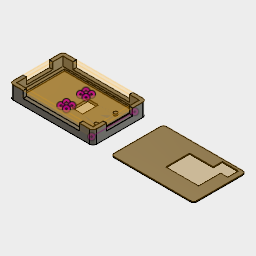
Tstat_case (Autodesk Fusion 360 design; units mm, degrees)
Autodesk Fusion 360 part; units mm, degrees
sketch "Sketch1" plane through (0, 0, 0) normal (0, 1, 0) x (1, 0, 0)
  line L0 (76, 53) -> (-76, 53)
  line L1 (-83, 46) -> (-83, -46)
  line L2 (-76, -53) -> (76, -53)
  line L3 (83, -46) -> (83, 46)
  line L4 (83, 53) -> (-83, -53) construction
  line L5 (-83, 53) -> (83, -53) construction
  line L6 (-76, 46) -> (76, 46)
  line L7 (76, 46) -> (76, -46)
  line L8 (76, -46) -> (-76, -46)
  line L9 (-76, -46) -> (-76, 46)
  line L10 (-76, 46) -> (76, -46) construction
  line L11 (76, 46) -> (-76, -46) construction
  arc A0 (-76, 53) -> (-83, 46) centre (-76, 46) ccw
  arc A1 (-83, -46) -> (-76, -53) centre (-76, -46) ccw
  arc A2 (83, 46) -> (76, 53) centre (76, 46) ccw
  arc A3 (76, -53) -> (83, -46) centre (76, -46) ccw
  dimension "d1" = 166
  dimension "d2" = 106
  dimension "d3" = 152
  dimension "d4" = 92
  dimension "d5" = 7
  dimension "d6" = 7
  dimension "d7" = 7
  dimension "d8" = 7
  constraint perpendicular L0 L1
  constraint parallel L0 L2
  constraint parallel L1 L3
  constraint horizontal L0
  constraint coincident L4
  constraint coincident L5
  constraint perpendicular L6 L7
  constraint parallel L6 L8
  constraint parallel L7 L9
  constraint horizontal L6
  constraint coincident L10
  constraint coincident L11
  constraint tangent L0 A0
  constraint tangent L1 A0
  constraint tangent L1 A1
  constraint tangent L2 A1
  constraint tangent L0 A2
  constraint tangent L3 A2
  constraint tangent L3 A3
  constraint tangent L2 A3
  measures "d5" radius of A0
  measures "d6" radius of A1
  measures "d7" radius of A2
  measures "d8" radius of A3
extrude "Extrude1" add sketch "Sketch1" along normal blind 5 contours L0 L1 L2 L3 A0 A1 A2 A3 | L6 L7 L8 L9 makes body 1
sketch "Sketch2" plane through (0, 5, 0) normal (0, 1, 0) x (-1, 0, 0)
  arc A0 (-76, 53) -> (-83, 46) centre (-76, 46) ccw
  line L0 (-83, 46) -> (-83, -46)
  arc A1 (-83, -46) -> (-76, -53) centre (-76, -46) ccw
  line L1 (-76, -53) -> (76, -53)
  arc A2 (76, -53) -> (83, -46) centre (76, -46) ccw
  line L2 (83, -46) -> (83, 46)
  arc A3 (83, 46) -> (76, 53) centre (76, 46) ccw
  line L3 (76, 53) -> (-76, 53)
  line L4 (-76, 46) -> (76, 46)
  line L5 (76, 46) -> (76, -46)
  line L6 (76, -46) -> (-76, -46)
  line L7 (-76, -46) -> (-76, 46)
  line L8 (-76, 46) -> (76, -46) construction
  line L9 (76, 46) -> (-76, -46) construction
  dimension "d11" = 152
  dimension "d12" = 92
  constraint perpendicular L4 L5
  constraint parallel L4 L6
  constraint parallel L5 L7
  constraint horizontal L4
  constraint coincident L8
  constraint coincident L9
extrude "Extrude2" add sketch "Sketch2" along normal blind 21.5 bodies 1
sketch "Sketch3" plane through (0, 5, 0) normal (0, 1, 0) x (-1, 0, 0)
  line L0 (76, -46) -> (76, 46)
  line L1 (76, 46) -> (-76, 46)
  line L2 (-76, 46) -> (-76, -46)
  line L3 (-76, -46) -> (76, -46)
  line L4 (70, -43) -> (-70, -43)
  line L5 (-70, -43) -> (-70, 43)
  line L6 (-70, 43) -> (70, 43)
  line L7 (70, 43) -> (70, -43)
  line L8 (70, -43) -> (-70, 43) construction
  line L9 (-70, -43) -> (70, 43) construction
  dimension "d15" = 140
  dimension "d16" = 86
  constraint perpendicular L4 L5
  constraint parallel L4 L6
  constraint parallel L5 L7
  constraint horizontal L4
  constraint coincident L8
  constraint coincident L9
extrude "Extrude3" add sketch "Sketch3" along normal blind 3.5 bodies 1
sketch "Sketch4" plane through (0, 5, 0) normal (0, 1, 0) x (-1, 0, 0)
  line L0 (-70, 43) -> (-70, -43)
  line L1 (-70, -43) -> (70, -43)
  line L2 (70, -43) -> (70, 43)
  line L3 (70, 43) -> (-70, 43)
  circle A0 centre (-55.85, -18.95) radius 3.45
  dimension "d19" = 6.9
  dimension "d20" = 14.15
  dimension "d21" = 24.05
  measures "d19" diameter of A0
  measures "d20" distance of L0
  measures "d21" distance of L1
extrude "Extrude4" add sketch "Sketch4" along normal blind 3.5 contours A0 bodies 1
sketch "Sketch5" plane through (0, 5, 0) normal (0, 1, 0) x (-1, 0, 0)
  circle A0 centre (-55.85, -18.95) radius 3.45
  line L0 (-70, 43) -> (-70, -43)
  line L1 (-70, -43) -> (70, -43)
  line L2 (70, -43) -> (70, 43)
  line L3 (70, 43) -> (-70, 43)
  line L4 (-1, -18.5) -> (-22, -18.5)
  line L5 (-22, -18.5) -> (-22, 12.5)
  line L6 (-22, 12.5) -> (-1, 12.5)
  line L7 (-1, 12.5) -> (-1, -18.5)
  line L8 (14, -30) -> (3, -30)
  line L9 (3, -30) -> (3, -19)
  line L10 (3, -19) -> (14, -19)
  line L11 (14, -19) -> (14, -30)
  line L12 (14, 9) -> (3, 9)
  line L13 (3, 9) -> (3, 20)
  line L14 (3, 20) -> (14, 20)
  line L15 (14, 20) -> (14, 9)
  dimension "d24" = 21
  dimension "d28" = 11
  dimension "d29" = 11
  dimension "d32" = 11
  dimension "d33" = 11
  dimension "d84" = 56
  dimension "d85" = 56
  dimension "d86" = 48
  dimension "d87" = 31
  dimension "d88" = 30.5
  dimension "d89" = 13
  dimension "d90" = 23
  constraint horizontal L4
  constraint vertical L5
  constraint horizontal L6
  constraint vertical L7
  constraint horizontal L8
  constraint vertical L9
  constraint horizontal L10
  constraint vertical L11
  constraint horizontal L12
  constraint vertical L13
  constraint horizontal L14
  constraint vertical L15
  measures "d84" distance of L2 L11
  measures "d85" distance of L2
  measures "d86" distance of L0 L5
  measures "d88" distance of L3 L6
  measures "d89" distance of L1
  measures "d90" distance of L3
extrude "Extrude5" cut sketch "Sketch5" against normal blind 5 contours L4 L5 L6 L7 bodies 1
extrude "Extrude11" add sketch "Sketch5" along normal blind 1 contours L8 L9 L10 L11 | L12 L13 L14 L15 bodies 1
sketch "Sketch6" plane through (0, 5, 0) normal (0, 1, 0) x (-1, 0, 0)
  line L0 (-22, -18.5) -> (-22, 12.5)
  line L1 (-22, 12.5) -> (-1, 12.5)
  line L2 (-1, 12.5) -> (-1, -18.5)
  line L3 (-1, -18.5) -> (-22, -18.5)
  circle A0 centre (-55.85, -18.95) radius 3.45
  line L4 (-70, 43) -> (-70, -43)
  line L5 (-70, -43) -> (70, -43)
  line L6 (70, -43) -> (70, 43)
  line L7 (70, 43) -> (-70, 43)
sketch "Sketch7" plane through (0, 5, 0) normal (0, 1, 0) x (-1, 0, 0)
  line L0 (-22, -18.5) -> (-22, 12.5)
  line L1 (-22, 12.5) -> (-1, 12.5)
  line L2 (-1, 12.5) -> (-1, -18.5)
  line L3 (-1, -18.5) -> (-22, -18.5)
  circle A0 centre (-55.85, -18.95) radius 3.45
  line L4 (-70, 43) -> (-70, -43)
  line L5 (-70, -43) -> (70, -43)
  line L6 (70, -43) -> (70, 43)
  line L7 (70, 43) -> (-70, 43)
sketch "Sketch8" plane through (0, 5, 0) normal (0, 1, 0) x (-1, 0, 0)
  line L0 (-22, -18.5) -> (-22, 12.5)
  line L1 (-22, 12.5) -> (-1, 12.5)
  line L2 (-1, 12.5) -> (-1, -18.5)
  line L3 (-1, -18.5) -> (-22, -18.5)
  circle A0 centre (-55.85, -18.95) radius 3.45
  line L4 (-70, 43) -> (-70, -43)
  line L5 (-70, -43) -> (70, -43)
  line L6 (70, -43) -> (70, 43)
  line L7 (70, 43) -> (-70, 43)
  circle A1 centre (-55.85, 18.95) radius 3.45
  dimension "d50" = 6.9
  dimension "d51" = 14.15
  dimension "d52" = 24.05
  measures "d50" diameter of A1
  measures "d51" distance of L4
  measures "d52" distance of L7
extrude "Extrude8" add sketch "Sketch8" along normal blind 3.5 contours A1 bodies 1
sketch "Sketch9" plane through (0, 5, 0) normal (0, 1, 0) x (-1, 0, 0)
  circle A0 centre (-55.85, 18.95) radius 3.45
  line L0 (-22, -18.5) -> (-22, 12.5)
  line L1 (-22, 12.5) -> (-1, 12.5)
  line L2 (-1, 12.5) -> (-1, -18.5)
  line L3 (-1, -18.5) -> (-22, -18.5)
  circle A1 centre (-55.85, -18.95) radius 3.45
  line L4 (-70, 43) -> (-70, -43)
  line L5 (-70, -43) -> (70, -43)
  line L6 (70, -43) -> (70, 43)
  line L7 (70, 43) -> (-70, 43)
  line L8 (14, 20) -> (14, 9)
  line L9 (14, 9) -> (3, 9)
  line L10 (3, 9) -> (3, 20)
  line L11 (3, 20) -> (14, 20)
  line L12 (14, -19) -> (14, -30)
  line L13 (14, -30) -> (3, -30)
  line L14 (3, -30) -> (3, -19)
  line L15 (3, -19) -> (14, -19)
sketch "Sketch10" plane through (0, 26.5, 0) normal (0, 1, 0) x (-1, 0, 0)
  line L0 (76, -46) -> (-76, -46)
  line L1 (-76, -46) -> (-76, 46)
  line L2 (-76, 46) -> (76, 46)
  line L3 (76, 46) -> (76, -46)
  line L4 (76, 53) -> (-76, 53)
  arc A0 (-76, 53) -> (-83, 46) centre (-76, 46) ccw
  line L5 (-83, 46) -> (-83, -46)
  arc A1 (-83, -46) -> (-76, -53) centre (-76, -46) ccw
  line L6 (-76, -53) -> (76, -53)
  arc A2 (76, -53) -> (83, -46) centre (76, -46) ccw
  line L7 (83, -46) -> (83, 46)
  arc A3 (83, 46) -> (76, 53) centre (76, 46) ccw
sketch "Sketch11" plane through (0, 26.5, 0) normal (0, 1, 0) x (-1, 0, 0)
  line L0 (-83, 26) -> (-76, 26)
  line L1 (-76, 26) -> (-76, -26)
  line L2 (-76, -26) -> (-83, -26)
  line L3 (-83, -26) -> (-83, 26)
  line L4 (-83, 46) -> (-83, -46)
  line L5 (-83, 46) -> (-83, -46)
  line L6 (76, 53) -> (-76, 53)
  line L7 (-56, 53) -> (56, 53)
  line L8 (56, 53) -> (56, 46)
  line L9 (56, 46) -> (-56, 46)
  line L10 (-56, 46) -> (-56, 53)
  line L11 (76, 26) -> (83, 26)
  line L12 (83, 26) -> (83, -26)
  line L13 (83, -26) -> (76, -26)
  line L14 (76, -26) -> (76, 26)
  line L15 (76, 46) -> (76, -46)
  line L16 (-56, -46) -> (56, -46)
  line L17 (56, -46) -> (56, -53)
  line L18 (56, -53) -> (-56, -53)
  line L19 (-56, -53) -> (-56, -46)
  line L20 (76, -46) -> (-76, -46)
  line L21 (76, -46) -> (-76, -46)
  dimension "d55" = 52
  dimension "d56" = 7
  dimension "d57" = 27
  dimension "d58" = 112
  dimension "d59" = 7
  dimension "d60" = 27
  dimension "d61" = 52
  dimension "d62" = 7
  dimension "d63" = 27
  dimension "d64" = 112
  dimension "d65" = 7
  dimension "d66" = 27
  constraint horizontal L0
  constraint vertical L1
  constraint horizontal L2
  constraint vertical L3
  constraint coincident L4
  constraint horizontal L7
  constraint vertical L8
  constraint horizontal L9
  constraint vertical L10
  constraint coincident L6
  constraint horizontal L11
  constraint vertical L12
  constraint horizontal L13
  constraint vertical L14
  constraint coincident L15
  constraint horizontal L16
  constraint vertical L17
  constraint horizontal L18
  constraint vertical L19
  constraint coincident L20
  measures "d57" distance of L0 L6
  measures "d60" distance of L10
  measures "d63" distance of L11
extrude "Extrude9" cut sketch "Sketch11" against normal blind 13.5 bodies 1
sketch "Sketch12" plane through (0, 0, 0) normal (0, 1, 0) x (1, 0, 0)
sketch "Sketch13" plane through (0, 0, 0) normal (0, 1, 0) x (1, 0, 0)
  line L0 (124, 52) -> (276, 52)
  line L1 (282, 46) -> (282, -46)
  line L2 (276, -52) -> (124, -52)
  line L3 (118, -46) -> (118, 46)
  line L4 (118.993, 51.3703) -> (282, -52) construction
  line L5 (283.3656, 54.353) -> (118.0012, -52.6297) construction
  arc A0 (124, 52) -> (118, 46) centre (124, 46) ccw
  arc A1 (118, -46) -> (124, -52) centre (124, -46) ccw
  arc A2 (282, 46) -> (276, 52) centre (276, 46) ccw
  line L6 (258, 29) -> (193, 29)
  line L7 (193, 29) -> (193, -18)
  line L8 (193, -18) -> (258, -18)
  line L9 (258, -18) -> (258, 29)
  line L10 (272, 47) -> (240, 47)
  line L11 (240, 47) -> (240, 26)
  line L12 (240, 26) -> (272, 26)
  line L13 (272, 26) -> (272, 47)
  arc A3 (276, -52) -> (282, -46) centre (276, -46) ccw
  dimension "d69" = 164
  dimension "d71" = 6
  dimension "d72" = 6
  dimension "d73" = 65
  dimension "d74" = 47
  dimension "d75" = 24
  dimension "d76" = 34
  dimension "d77" = 32
  dimension "d79" = 5
  dimension "d80" = 10
  dimension "d81" = 6
  dimension "d93" = 104
  dimension "d94" = 21
  constraint perpendicular L0 L1
  constraint parallel L0 L2
  constraint parallel L1 L3
  constraint horizontal L0
  constraint coincident L4
  constraint coincident L5
  constraint tangent L0 A0
  constraint tangent L3 A0
  constraint tangent L3 A1
  constraint tangent L2 A1
  constraint tangent L1 A2
  constraint tangent L0 A2
  constraint equal A1 A2
  constraint horizontal L6
  constraint vertical L7
  constraint horizontal L8
  constraint vertical L9
  constraint horizontal L10
  constraint vertical L11
  constraint horizontal L12
  constraint vertical L13
  constraint tangent L2 A3
  constraint tangent L1 A3
  measures "d71" radius of A0
  measures "d72" radius of A1
  measures "d75" distance of L1 L9
  measures "d76" distance of L2 L8
  measures "d79" distance of L0 L10
  measures "d80" distance of L1 L13
  measures "d81" radius of A3
extrude "Extrude10" add sketch "Sketch13" along normal blind 2 separate body makes body 2
sketch "Sketch14" plane through (0, 2, 0) normal (0, 1, 0) x (-1, 0, 0)
  line L0 (-272, -47) -> (-272, -26)
  line L1 (-272, -26) -> (-258, -26)
  line L2 (-258, -26) -> (-258, 18)
  line L3 (-258, 18) -> (-193, 18)
  line L4 (-193, 18) -> (-193, -29)
  line L5 (-193, -29) -> (-240, -29)
  line L6 (-240, -29) -> (-240, -47)
  line L7 (-240, -47) -> (-272, -47)
  arc A0 (-118, 46) -> (-124, 52) centre (-124, 46) ccw
  line L8 (-124, 52) -> (-276, 52)
  arc A1 (-276, 52) -> (-282, 46) centre (-276, 46) ccw
  line L9 (-282, 46) -> (-282, -46)
  arc A2 (-282, -46) -> (-276, -52) centre (-276, -46) ccw
  line L10 (-276, -52) -> (-124, -52)
  arc A3 (-124, -52) -> (-118, -46) centre (-124, -46) ccw
  line L11 (-118, -46) -> (-118, 46)
